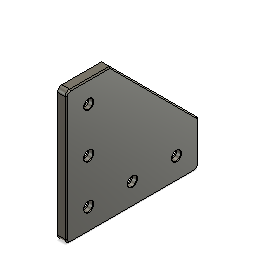
40x40_bracket (Autodesk Fusion 360 design; units mm, degrees)
Autodesk Fusion 360 part; units mm, degrees
note: some values were not read from the file. Chosen so that the rebuilt part matches the saved one: which face or edge a step refers to.
sketch "Sketch1" plane through (0, 0, 0) normal (1, 0, 0) x (0, 0, -1)
  line L0 (0, 0) -> (0, -60)
  line L1 (0, -60) -> (60, -60)
  line L2 (60, -60) -> (60, -40)
  line L3 (20, 0) -> (0, 0)
  line L4 (60, -40) -> (40, -20)
  line L5 (60, -50) -> (0, -50) construction
  line L6 (10.2088, 0) -> (10.2088, -60) construction
  line L7 (0, -9.7462) -> (40, -10) construction
  line L8 (0, -30) -> (50, -30) construction
  line L9 (49.9986, -60) -> (50, -30) construction
  line L10 (30, -60) -> (30, 0) construction
  circle A0 centre (10.2088, -9.811) radius 2.1
  circle A1 centre (10.2088, -30) radius 2.1
  circle A2 centre (10.2088, -50) radius 2.1
  circle A3 centre (30, -50) radius 2.1
  circle A4 centre (49.9991, -50) radius 2.1
  line L11 (60, -40) -> (20, 0)
  dimension "d1" = 60
  dimension "d2" = 60
  dimension "d3" = 20
  dimension "d15" = 4.2
  dimension "d16" = 4.2
  dimension "d17" = 4.2
  dimension "d18" = 4.2
  dimension "d19" = 4.2
  constraint coincident L0.start L3.end
  constraint vertical L0
  constraint perpendicular L0 L1
  constraint perpendicular L1 L2
  constraint perpendicular L0 L3
  constraint midpoint L2 L5.start
  constraint coincident L0 L5.end
  constraint perpendicular L0 L5
  constraint coincident L3 L6.start
  constraint coincident L1 L6.end
  constraint perpendicular L1 L6
  constraint coincident L0 L7.start
  constraint midpoint L0 L8.start
  constraint midpoint L4 L8.end
  constraint perpendicular L0 L8
  constraint coincident L1 L9.start
  constraint midpoint L1 L10.start
  constraint coincident L3 L10.end
  constraint perpendicular L3 L10
  constraint coincident L7 A0.centre
  constraint coincident L6 A0.centre
  constraint midpoint L6 A1.centre
  constraint coincident L5 A2.centre
  constraint coincident L6 A2.centre
  constraint midpoint L5 A3.centre
  constraint coincident L5 A4.centre
  constraint coincident L9 A4.centre
  constraint parallel L4 L11
  measures "d1" distance of L0.start L0.end
  measures "d2" distance of L0.end L1.end
  measures "d3" distance of L1.end L2.end
  measures "d15" diameter of A0
  measures "d16" diameter of A1
  measures "d17" diameter of A2
  measures "d18" diameter of A3
  measures "d19" diameter of A4
extrude "Extrude1" add sketch "Sketch1" along normal blind 4
chamfer "Chamfer1" distance 2 angle 45 5 edges at (0, -9.0516, -8.2509) (0, -29.2406, -8.2509) (0, -49.2406, -8.2509) (0, -49.2406, -28.0421) (0, -49.2406, -48.0412)
fillet "Fillet1" radius 2 4 edges at (2, -60, -60) (2, -60, 0) (2, -40, -60) (2, 0, 0)
chamfer "Chamfer2" distance 0.5 angle 45 9 edges at (4, 0, -11) (4, -0.5858, -0.5858) (4, -19.7071, -39.7071) (4, -30, 0) (4, -40.0631, -59.8478) (4, -59.4142, -0.5858) (4, -49.4142, -60) (4, -60, -30) (4, -59.4142, -59.4142)
chamfer "Chamfer3" distance 0.2 angle 45 5 edges at (4, -9.0516, -8.2509) (4, -29.2406, -8.2509) (4, -49.2406, -8.2509) (4, -49.2406, -28.0421) (4, -49.2406, -48.0412)
